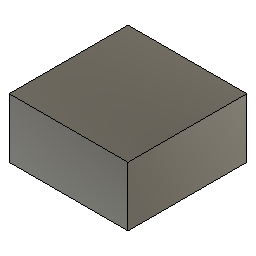
Flat keycap v2 (Autodesk Fusion 360 design; units mm, degrees)
Autodesk Fusion 360 part; units mm, degrees
note: some values were not read from the file. Chosen so that the rebuilt part matches the saved one: where a step ends; a direction.
sketch "Sketch8" plane through (0, 0, 0) normal (0, 0, 1) x (1, 0, 0)
  circle A0 centre (25.55, 0.35) radius 2.75
  line L0 (25, -1.7) -> (26.24, -1.7)
  line L1 (26.1002, 2.4) -> (25, 2.4)
  line L2 (27.6, -0.2) -> (27.6, 1.0403)
  line L3 (23.5, 1.04) -> (23.5, -0.2)
  line L4 (25, -1.7) -> (25, -0.5)
  line L5 (23.5, 1.04) -> (24.7, 1.04)
  line L6 (25, 1.34) -> (25, 2.54)
  line L7 (23.5, -0.2) -> (24.7, -0.2)
  line L8 (26.24, -1.7) -> (26.24, -0.5)
  line L9 (26.54, -0.2) -> (27.6, -0.2)
  line L10 (27.6, 1.0403) -> (26.4, 1.0403)
  line L11 (26.1, 1.3404) -> (26.1002, 2.4)
  arc A1 (25, -0.5) -> (24.7, -0.2) centre (24.7, -0.5) ccw
  arc A2 (26.54, -0.2) -> (26.24, -0.5) centre (26.54, -0.5) ccw
  arc A3 (26.1, 1.3404) -> (26.4, 1.0403) centre (26.4, 1.3403) ccw
  arc A4 (24.7, 1.04) -> (25, 1.34) centre (24.7, 1.34) ccw
  point P0 (25, -0.2)
  point P1 (25, 1.04)
  point P2 (26.24, -0.2)
  point P3 (26.1, 1.0403)
  dimension "d42" = 5.5
  dimension "d47" = 1.24
  dimension "d48" = 4.1
  dimension "d50" = 4.1
  dimension "d51" = 1.24
  dimension "d53" = 1.5
  dimension "d54" = 1.5
  dimension "d55" = 1.5
  dimension "d56" = 1.5
  dimension "d57" = 1.5
  dimension "d58" = 0.3
  dimension "d59" = 0.3
  dimension "d60" = 0.3
  dimension "d61" = 0.3
  dimension "d67" = 2.05
  dimension "d68" = 2.05
  constraint horizontal L0
  constraint horizontal L1
  constraint vertical L2
  constraint vertical L3
  constraint perpendicular L0 L4
  constraint horizontal L5
  constraint vertical L6
  constraint perpendicular L4 L7
  constraint perpendicular L0 L8
  constraint perpendicular L2 L9
  constraint horizontal L10
  constraint coincident P0 L7
  constraint coincident P0 L4
  constraint tangent L7 A1
  constraint tangent L4 A1
  constraint coincident P2 L8
  constraint coincident P2 L9
  constraint tangent L8 A2
  constraint tangent L9 A2
  constraint coincident P3 L11
  constraint coincident P3 L10
  constraint tangent L11 A3
  constraint tangent L10 A3
  constraint coincident P1 L5
  constraint coincident P1 L6
  constraint tangent L5 A4
  constraint tangent L6 A4
  measures "d42" diameter of A0
  measures "d47" distance of L0.start L0.end
  measures "d48" distance of L0.start L1.end
  measures "d50" distance of L3.end L2.start
  measures "d51" distance of L3.end L3.start
  measures "d53" distance of L0.start P0
  measures "d54" distance of L3.start P1
  measures "d55" distance of P1 L6.end
  measures "d56" distance of L0.end P2
  measures "d57" distance of L2.end P3
  measures "d58" radius of A1
  measures "d59" radius of A2
  measures "d60" radius of A3
  measures "d61" radius of A4
  measures "d67" distance of A0.centre L0
  measures "d68" distance of A0.centre L2
extrude "Extrude5" add sketch "Sketch8" along normal blind 6 makes body 1
chamfer "Chamfer2" distance 0.25 angle 45 16 edges at (25, -1.1, 0) (24.9121, -0.2879, 0) (24.1, -0.2, 0) (26.24, -1.1, 0) (27.07, -0.2, 0) (26.3279, -0.2879, 0) (27, 1.0403, 0) (26.1001, 1.8702, 0) (26.1879, 1.1282, 0) (24.9121, 1.1279, 0) (25, 1.87, 0) (24.1, 1.04, 0) (23.5, 0.42, 0) (25.62, -1.7, 0) (27.6, 0.4202, 0) (25.5501, 2.4, 0) on bodies 1
sketch "Sketch9" plane through (0, 0, 6) normal (0, 0, 1) x (-1, 0, 0)
  line L0 (-23.5, 0.2) -> (-23.5, -1.04)
  line L1 (-23.5, -1.04) -> (-24.7, -1.04)
  arc A0 (-24.7, -1.04) -> (-25, -1.34) centre (-24.7, -1.34) ccw
  line L2 (-25, -1.34) -> (-25, -2.4)
  line L3 (-25, -2.4) -> (-26.1002, -2.4)
  line L4 (-26.1002, -2.4) -> (-26.1, -1.3404)
  arc A1 (-26.1, -1.3404) -> (-26.4, -1.0403) centre (-26.4, -1.3403) ccw
  line L5 (-26.4, -1.0403) -> (-27.6, -1.0403)
  line L6 (-27.6, -1.0403) -> (-27.6, 0.2)
  line L7 (-27.6, 0.2) -> (-26.54, 0.2)
  arc A2 (-26.54, 0.2) -> (-26.24, 0.5) centre (-26.54, 0.5) ccw
  line L8 (-26.24, 0.5) -> (-26.24, 1.7)
  line L9 (-26.24, 1.7) -> (-25, 1.7)
  line L10 (-25, 1.7) -> (-25, 0.5)
  arc A3 (-25, 0.5) -> (-24.7, 0.2) centre (-24.7, 0.5) ccw
  line L11 (-24.7, 0.2) -> (-23.5, 0.2)
  circle A4 centre (-25.55, -0.35) radius 2.75
  line L12 (-16.55, -9.35) -> (-34.55, -9.35)
  line L13 (-34.55, -9.35) -> (-34.55, 8.65)
  line L14 (-34.55, 8.65) -> (-16.55, 8.65)
  line L15 (-16.55, 8.65) -> (-16.55, -9.35)
  line L16 (-16.55, -9.35) -> (-34.55, 8.65) construction
  line L17 (-34.55, -9.35) -> (-16.55, 8.65) construction
  line L18 (-25.55, -3.1) -> (-25.55, -9.35)
  line L19 (-22.8, -0.35) -> (-16.55, -0.35)
  line L20 (-23.6055, -2.2945) -> (-16.55, -9.35)
  line L21 (-27.4945, -2.2945) -> (-34.55, -9.35)
  line L22 (-27.4945, 1.5945) -> (-34.55, 8.65)
  line L23 (-23.6055, 1.5945) -> (-16.55, 8.65)
  line L24 (-25.55, 2.4) -> (-25.55, 8.65)
  line L25 (-28.3, -0.35) -> (-34.55, -0.35)
  circle A5 centre (-25.55, -0.35) radius 4.75
  point P0 (-25.55, -0.35)
  dimension "d69" = 18
  dimension "d70" = 18
  dimension "d79" = 9.5
  constraint horizontal L12
  constraint perpendicular L12 L13
  constraint parallel L12 L14
  constraint parallel L13 L15
  constraint coincident L16 P0
  constraint coincident L17 P0
  constraint coincident P0 A4.centre
  constraint coincident A4 L18.start
  constraint midpoint L12 L18.end
  constraint perpendicular L12 L18
  constraint coincident A4 L19.start
  constraint midpoint L15 L19.end
  constraint perpendicular L15 L19
  constraint coincident L16 L20.start
  constraint coincident A4 L20.start
  constraint coincident L17 L21.start
  constraint coincident A4 L21.start
  constraint coincident A4 L22.start
  constraint coincident L16 L22.start
  constraint coincident L17 L23.start
  constraint coincident A4 L23.start
  constraint coincident A4 L24.start
  constraint midpoint L14 L24.end
  constraint perpendicular L14 L24
  constraint coincident A4 L25.start
  constraint midpoint L13 L25.end
  constraint perpendicular L13 L25
  measures "d69" distance of L13.end L14.end
  measures "d70" distance of L12.end L13.end
  measures "d79" diameter of A5
extrude "Extrude7" add sketch "Sketch9" along normal blind 2 separate body contours L0 L1 A0 L2 L3 L4 A1 L5 L6 L7 A2 L8 L9 L10 A3 L11 | A4 | A4 L19 L20 A5 | A4 L19 L23 A5 | A4 L23 L24 A5 | A4 L18 L20 A5 | L15 L19 L23 A5 | L15 L19 L20 A5 | A4 L22 L24 A5 | L14 L23 L24 A5 | A4 L18 L21 A5 | L12 L18 L20 A5 | A4 L22 L25 A5 | L14 L22 L24 A5 | A4 L21 L25 A5 | L12 L18 L21 A5 | L13 L22 L25 A5 | L13 L21 L25 A5 makes body 2
extrude "Extrude8" add sketch "Sketch9" against normal blind 6 contours A4 L19 L20 A5 | A4 L19 L23 A5 | A4 L23 L24 A5 | A4 L18 L20 A5 | L15 L19 L23 A5 | L15 L19 L20 A5 | A4 L22 L24 A5 | L14 L23 L24 A5 | A4 L18 L21 A5 | L12 L18 L20 A5 | A4 L22 L25 A5 | L14 L22 L24 A5 | A4 L21 L25 A5 | L12 L18 L21 A5 | L13 L22 L25 A5 | L13 L21 L25 A5 bodies 2
shell "Shell2" thickness 1.2 removed faces 1 at (25.6185, -6.5641, 0) on bodies 2
delete_face "DeleteFace1" 1 faces at (21.6049, 0.5469, 2.2667) on bodies 2
rib "Web2" add thickness 0.6 on both sides direction (0, 0, -1) depth 2.7 path "Sketch9" along L23 L24 L22 L25 L21 L18 L20 L19 A5 bodies 2
sketch "Sketch11" plane through (0, 0, 8) normal (0, 0, 1) x (-1, 0, 0)
  line L0 (-16.55, 8.65) -> (-34.55, 8.65)
  line L1 (-34.55, 8.65) -> (-34.55, -9.35)
  line L2 (-34.55, -9.35) -> (-16.55, -9.35)
  line L3 (-16.55, -9.35) -> (-16.55, 8.65)
extrude "Extrude9" add 1 faces at (22.55, -2.65, 8) along direction (0, 0, 1) blind 1 on bodies 2 bodies 2
sketch "Sketch12" plane through (0, 0, 9) normal (0, 0, 1) x (-1, 0, 0)
  line L0 (-16.55, 8.65) -> (-34.55, 8.65)
  line L1 (-34.55, 8.65) -> (-34.55, -9.35)
  line L2 (-34.55, -9.35) -> (-16.55, -9.35)
  line L3 (-16.55, -9.35) -> (-16.55, 8.65)
named bodies: "center", "top"
